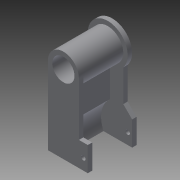
# Autodesk Inventor part: tendeur
Saved by Autodesk Inventor 2015 (Build 190159000, 159)
## iProperties
Created: 2015-09-12
Part Number: tendeur
Material: Générique
Document SubType Name: Modeling
Designer: astralien3000
Density: 1 g/cm^3
Appearance: Par défaut
Author: astralien3000
Autodesk Inventor part; units mm, degrees
ref_plane "YZ Plane" through (0, 0, 0) normal (1, 0, 0) x (0, 1, 0)
ref_plane "XZ Plane" through (0, 0, 0) normal (0, 1, 0) x (-1, 0, 0)
ref_plane "XY Plane" through (0, 0, 0) normal (0, 0, 1) x (1, 0, 0)
sketch "Esquisse1" plane through (0, 0, 0) normal (0, 1, 0) x (-1, 0, 0)
  arc A0 (-0.5, -2.4495) -> (0.5, -2.4495) centre (0, 0) ccw
  arc A1 (0.5, -3.4641) -> (-0.5, -3.4641) centre (0, 0) ccw
  arc A2 (0.5, -11.6834) -> (-0.5, -10.5279) centre (-4.5, -15) ccw
  arc A3 (0.5, -10.101) -> (-0.5, -9.2554) centre (-4.5, -15) ccw
  line L0 (-11.5, 3.5) -> (3.5, 3.5)
  line L1 (3.5, 3.5) -> (3.5, -17.5)
  line L2 (3.5, -17.5) -> (2.0383, -17.5)
  line L3 (-11.5, -17.5) -> (-11.5, 3.5)
  line L4 (-0.5, 0) -> (0.5, 0)
  line L5 (0.5, 0) -> (0.5, -2.4495)
  line L6 (0.5, -15) -> (-0.5, -15)
  line L7 (-0.5, -15) -> (-0.5, -10.5279)
  line L8 (0.5, -10.101) -> (0.5, -15)
  line L9 (-0.5, -9.2554) -> (-0.5, -3.4641)
  arc A4 (2.0383, -17.5) -> (0.5, -10.101) centre (-4.5, -15) ccw
  arc A5 (0.9544, -17.5) -> (0.5, -11.6834) centre (-4.5, -15) ccw
  line L10 (2.0383, -17.5) -> (0.9544, -17.5)
  line L11 (0.9544, -17.5) -> (-11.5, -17.5)
  arc A6 (-0.5, -10.5279) -> (0.9544, -17.5) centre (-4.5, -15) ccw
  arc A7 (-0.5, -9.2554) -> (2.0383, -17.5) centre (-4.5, -15) ccw
  line L12 (-0.5, -10.5279) -> (-0.5, -9.2554)
  arc A8 (0.5, -2.4495) -> (-0.5, -2.4495) centre (0, 0) ccw
  arc A9 (-0.5, -3.4641) -> (0.5, -3.4641) centre (0, 0) ccw
  line L13 (-0.5, -3.4641) -> (-0.5, -2.4495)
  line L14 (0.5, -2.4495) -> (0.5, -3.4641)
  line L15 (0.5, -3.4641) -> (0.5, -10.101)
  line L16 (-0.5, -2.4495) -> (-0.5, 0)
  dimension "d0" = 5
  dimension "d1" = 1
  dimension "d2" = 14
  dimension "d3" = 1
  dimension "d4" = 15
  dimension "d6" = 8
  dimension "d7" = 21
  dimension "d9" = 1
  dimension "d10" = 0.5
  constraints: 34 end point, 25 parallel, 20 point on circle, 10 centre point, 5 perpendicular, 5 point on line, 4 tangent, 3 coincident, 2 horizontal, 1 midpoint
  measures "d0" diameter of A0
  measures "d1" radial gap between concentric circles of A1 A0
  measures "d2" diameter of A3
  measures "d3" radial gap between concentric circles of A3 A2
  measures "d4" vertical distance of point (0, 0) A2.centre
  measures "d6" distance from line of L1 A2.centre
  measures "d7" distance between parallel lines of L0 L2
  measures "d9" distance between parallel lines of L7 L5
  measures "d10" distance from line of L5 point (0, 0)
extrude "Extrusion1" add sketch "Esquisse1" against normal blind 9 contours L13 A1 L14 A8 | A9 L15 A3 L9 | A3 L8 A2 L12 | A4 L10 A5 L8
sketch "Esquisse2" plane through (0, 0, 0) normal (0, 1, 0) x (1, 0, 0)
  line L0 (0.5, 3.4641) -> (0.5, 2.4495) projected
  arc A0 (-0.5, 2.4495) -> (0.5, 2.4495) centre (0, 0) ccw projected
  line L1 (-0.5, 2.4495) -> (-0.5, 3.4641) projected
  arc A1 (-0.5, 2.4495) -> (0.5, 2.4495) centre (0, 0) ccw
  arc A2 (-0.5, 3.4641) -> (0.5, 3.4641) centre (0, 0) ccw
  arc A3 (0.5, 2.4495) -> (-0.5, 2.4495) centre (0, 0) ccw
  arc A4 (0.5, 3.4641) -> (-0.5, 3.4641) centre (0, 0) ccw
  constraints: 8 point on circle, 4 centre point, 4 end point, 2 coincident
extrude "Extrusion2" add sketch "Esquisse2" against normal blind 9 contours L0 A3 L1 A4
sketch "Esquisse3" plane through (0, 0, 0) normal (0, 1, 0) x (1, 0, 0)
  circle A0 centre (0, 0) radius 2.5 projected
  arc A1 (-0.9544, 17.5) -> (0.5, 10.5279) centre (4.5, 15) ccw projected
  line L0 (-0.9544, 17.5) -> (-2.0383, 17.5) projected
  arc A2 (-0.5, 3.4641) -> (0.5, 3.4641) centre (0, 0) ccw projected
  line L1 (5.5, 17.5) -> (-4.5, 17.5)
  line L2 (-4.5, 17.5) -> (-4.5, 12)
  line L3 (-4.5, 12) -> (5.5, 12)
  line L4 (5.5, 12) -> (5.5, 17.5)
  arc A3 (3.5, 2.8284) -> (-4.5, 0) centre (0, 0) ccw
  line L5 (-4.5, 0) -> (-2.5, 0)
  line L6 (3.5, 0) -> (3.5, 2.8284)
  line L7 (3.5, 12) -> (-4.5, 12)
  line L8 (-4.5, 12) -> (-4.5, 0)
  line L9 (5.5, 12) -> (3.5, 10)
  line L10 (3.5, 2.8284) -> (3.5, 12)
  arc A4 (-4.5, 0) -> (3.5, 2.8284) centre (0, 0) ccw
  arc A5 (2.5, 0) -> (-2.5, 0) centre (0, 0) ccw
  line L11 (2.5, 0) -> (3.5, 0)
  line L12 (-2.5, 0) -> (2.5, 0)
  arc A6 (-2.5, 0) -> (2.5, 0) centre (0, 0) ccw
  dimension "d15" = 1
  dimension "d16" = 3
  dimension "d18" = 1
  dimension "d19" = 8
  dimension "d20" = 135
  constraints: 24 end point, 8 point on circle, 7 parallel, 7 perpendicular, 4 centre point, 4 horizontal, 3 point on line, 2 coincident, 1 collinear, 1 horizontal alignment, 1 tangent, 2 other
  measures "d15" distance from line of A1.centre L4
  measures "d16" distance from line of L3 A1.centre
  measures "d18" radial gap between concentric circles of A3 A2
  measures "d19" distance between parallel lines of L8 L6
  measures "d20" angle of L3 L9
extrude "Extrusion3" add sketch "Esquisse3" along normal blind 1 contours L11 A2 L5 A0 | A0 L5 A3 L6 L11 | L6 A4 L5 A2 | A3 L8 L3 L10 | L10 L3 L9 | L2 L1 L0 A1 L3 | L3 A1 L1 L4
sketch "Esquisse4" plane through (0, -9, 0) normal (0, -1, 0) x (1, 0, 0)
  arc A0 (0.5, -3.4641) -> (-0.5, -3.4641) centre (0, 0) ccw projected
  line L0 (-0.5, -3.4641) -> (-0.5, -10.101) projected
  line L1 (-2.0383, -17.5) -> (-0.9544, -17.5) projected
  line L2 (0.5, -10.5279) -> (0.5, -3.4641) projected
  circle A1 centre (0, 0) radius 2.5 projected
  line L3 (-3.5, 0) -> (-2.5, 0)
  line L4 (3.5, 0) -> (3.5, -10)
  line L5 (3.5, -17.5) -> (-3.5, -17.5)
  line L6 (-3.5, -17.5) -> (-3.5, 0)
  arc A2 (3.5, 0) -> (-3.5, 0) centre (0, 0) ccw
  arc A3 (-2.5, 0) -> (2.5, 0) centre (0, 0) ccw
  line L7 (3.5, -17.5) -> (5.5, -17.5)
  line L8 (5.5, -17.5) -> (5.5, -12)
  line L9 (5.5, -12) -> (3.5, -12)
  line L10 (3.5, -12) -> (3.5, -17.5)
  line L11 (5.5, -12) -> (3.5, -12)
  line L12 (3.5, -12) -> (3.5, -10)
  line L13 (3.5, -10) -> (5.5, -10)
  line L14 (5.5, -10) -> (5.5, -12)
  arc A4 (0.5, -3.4641) -> (3.5, 0) centre (0, 0) ccw
  arc A5 (-0.5, -3.4641) -> (0.5, -3.4641) centre (0, 0) ccw
  arc A6 (-3.5, 0) -> (-0.5, -3.4641) centre (0, 0) ccw
  arc A7 (2.5, 0) -> (-2.5, 0) centre (0, 0) ccw
  line L15 (2.5, 0) -> (3.5, 0)
  line L16 (-2.5, 0) -> (2.5, 0)
  line L17 (3.5, -10) -> (3.5, -12)
  line L18 (3.5, -12) -> (3.5, -17.5)
  line L19 (3.5, -10) -> (5.5, -12)
  constraints: 36 end point, 13 point on circle, 11 perpendicular, 10 parallel, 6 centre point, 5 horizontal, 4 coincident, 3 tangent, 2 concentric, 1 collinear, 1 point on line
extrude "Extrusion4" add sketch "Esquisse4" along normal blind 1 contours A5 A0 L3 A1 L15 | A0 L4 L12 L10 L5 L1 L6 A5 | L15 A1 L3 A0 | L9 L8 L7 L10
sketch "Esquisse5" plane through (0, 0, 0) normal (0, -1, 0) x (1, 0, 0)
  arc A0 (-0.5, -10.101) -> (-2.0383, -17.5) centre (4.5, -15) ccw projected
  circle A1 centre (4.5, -15) radius 0.5
  dimension "d25" = 1
  constraints: 1 centre point, 1 coincident
  measures "d25" diameter of A1
extrude "Extrusion5" cut sketch "Esquisse5" along normal through all both and the other way through all
